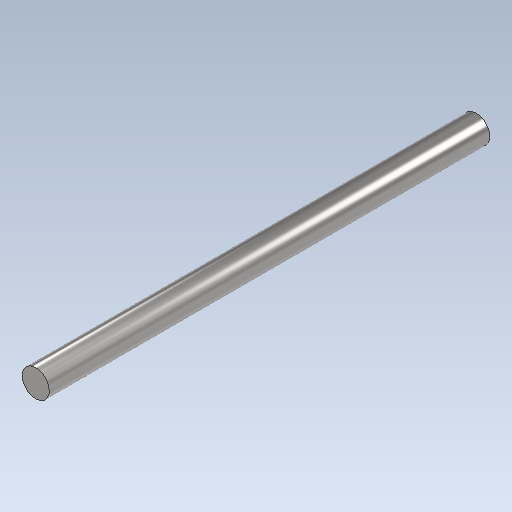
# Autodesk Inventor part: shaft
Saved by Autodesk Inventor 2021.1 (Build 251245010, 245A)
## iProperties
Created: 2023-03-23
Part Number: shaft
Material: Steel, Alloy
Document SubType Name: Modeling
Designer: M
Density: 7.73 g/cm^3
Appearance: Semi-Polished
Mass: 130.554 g
Surface Area: 85.4513 cm^2
Volume: 16.8892 cm^3
Author: M
Autodesk Inventor part; units mm, degrees
note: some values were not read from the file. Chosen so that the rebuilt part matches the saved one: second side of "Extrusion1".
ref_plane "YZ Plane" through (0, 0, 0) normal (1, 0, 0) x (0, 1, 0)
ref_plane "XZ Plane" through (0, 0, 0) normal (0, 1, 0) x (-1, 0, 0)
ref_plane "XY Plane" through (0, 0, 0) normal (0, 0, 1) x (1, 0, 0)
sketch "Sketch1" plane through (0, 0, 0) normal (0, 0, 1) x (1, 0, 0)
  arc A0 (-17.6547, 8.7) -> (-17.6547, 9.9) centre (-13.7, 9.3) ccw projected
  circle A1 centre (-13.7, 9.3) radius 4
  point P0 (0, 0)
  constraints: 1 centre point, 1 coincident, 1 concentric
extrude "Extrusion1" add sketch "Sketch1" against normal blind 130
body "Solid1"
